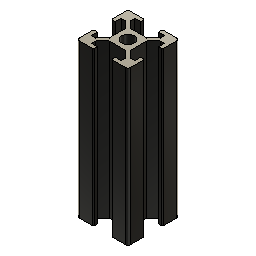
Support_Arm_ Assembly v9 (Autodesk Fusion 360 archive; units mm, degrees)
design "2020 Extrusion 60mm"
Autodesk Fusion 360 part; units mm, degrees
sketch "Sketch1" plane through (0, 0, 0) normal (0, 0, 1) x (1, 0, 0)
  line L0 (0, 1) -> (0, 6.1503)
  line L1 (1, 0) -> (6.15, 0)
  line L2 (0.3536, 6.5038) -> (1.5038, 6.5038)
  line L3 (1.5038, 6.5038) -> (1.5038, 4.2038)
  line L4 (1.5038, 4.2038) -> (3.2139, 4.2038)
  line L5 (3.2139, 4.2038) -> (5.804, 6.7939)
  line L6 (6.5036, 0.3536) -> (6.5036, 1.5036)
  line L7 (6.5036, 1.5036) -> (4.2036, 1.5036)
  line L8 (4.2036, 1.5036) -> (4.2036, 3.2136)
  line L9 (4.2036, 3.2136) -> (6.7937, 5.8037)
  line L10 (0, 6.1503) -> (0.3536, 6.5038)
  line L11 (6.15, 0) -> (6.5036, 0.3536)
  circle A0 centre (10, 10) radius 2.45
  line L12 (10, 10) -> (0, 0) construction
  line L13 (0, 19) -> (0, 13.85)
  line L14 (1, 20) -> (6.15, 20)
  line L15 (0, 13.85) -> (0.3536, 13.4964)
  line L16 (0, 13.85) -> (0.5, 13.85) construction
  line L17 (0.3536, 13.4964) -> (1.5036, 13.4964)
  line L18 (1.5036, 13.4964) -> (1.5036, 15.7964)
  line L19 (0, 20) -> (10, 10) construction
  line L20 (5.804, 6.7939) -> (5.804, 13.2061)
  line L21 (5.804, 13.2061) -> (3.2139, 15.7962)
  line L22 (1.5036, 15.7964) -> (3.2139, 15.7962)
  line L23 (6.15, 20) -> (6.5036, 19.6464)
  line L24 (6.15, 20) -> (6.65, 20) construction
  line L25 (6.5036, 19.6464) -> (6.5036, 18.4964)
  line L26 (6.5036, 18.4964) -> (4.2036, 18.4964)
  line L27 (4.2036, 18.4964) -> (4.2036, 16.7864)
  line L28 (4.2036, 16.7864) -> (6.7937, 14.1963)
  line L29 (10, 10) -> (20, 20) construction
  line L30 (10, 10) -> (20, 0) construction
  line L31 (19, 20) -> (13.85, 20)
  line L32 (20, 19) -> (20, 13.85)
  line L33 (13.85, 20) -> (13.4964, 19.6464)
  line L34 (13.85, 20) -> (14.35, 20) construction
  line L35 (13.4964, 19.6464) -> (13.4964, 18.4964)
  line L36 (20, 13.85) -> (19.6464, 13.4964)
  line L37 (20, 13.85) -> (20.5, 13.85) construction
  line L38 (19.6464, 13.4964) -> (18.4964, 13.4964)
  line L39 (13.4964, 18.4964) -> (15.7964, 18.4964)
  line L40 (18.4964, 13.4964) -> (18.4964, 15.7964)
  line L41 (15.7964, 18.4964) -> (15.7964, 16.7864)
  line L42 (15.7964, 16.7864) -> (13.2064, 14.1963)
  line L43 (13.2064, 14.1963) -> (6.7937, 14.1963)
  line L44 (18.4964, 15.7964) -> (16.7864, 15.7964)
  line L45 (16.7864, 15.7964) -> (14.1963, 13.2063)
  line L46 (19, 0) -> (13.85, 0)
  line L47 (20, 1) -> (20, 6.15)
  line L48 (13.85, 0) -> (13.4964, 0.3536)
  line L49 (13.85, 0) -> (14.35, 0) construction
  line L50 (13.4964, 0.3536) -> (13.4964, 1.5036)
  line L51 (13.4964, 1.5036) -> (15.7964, 1.5036)
  line L52 (15.7964, 1.5036) -> (15.7964, 3.2136)
  line L53 (15.7964, 3.2136) -> (13.2063, 5.8037)
  line L54 (6.7937, 5.8037) -> (13.2063, 5.8037)
  line L55 (20, 6.15) -> (19.6464, 6.5036)
  line L56 (20, 6.15) -> (20.5, 6.15) construction
  line L57 (19.6464, 6.5036) -> (18.4964, 6.5036)
  line L58 (18.4964, 6.5036) -> (18.4964, 4.2036)
  line L59 (18.4964, 4.2036) -> (16.7864, 4.2036)
  line L60 (16.7864, 4.2036) -> (14.1963, 6.7937)
  line L61 (14.1963, 6.7937) -> (14.1963, 13.2063)
  arc A1 (0, 1) -> (1, 0) centre (1, 1) ccw
  arc A2 (1, 20) -> (0, 19) centre (1, 19) ccw
  arc A3 (20, 19) -> (19, 20) centre (19, 19) ccw
  arc A4 (19, 0) -> (20, 1) centre (19, 1) ccw
  dimension "d9" = 2.3
  dimension "d11" = 3.663
  dimension "d13" = 2.3
  dimension "d17" = 135
  dimension "d18" = 135
  dimension "d19" = 135
  dimension "d20" = 6.1503
  dimension "d21" = 1.1503
  dimension "d22" = 0.5
  dimension "d23" = 135
  dimension "d24" = 0.5
  dimension "d25" = 6.15
  dimension "d26" = 1.15
  dimension "d27" = 4.9
  dimension "d28" = 10
  dimension "d29" = 10
  dimension "d30" = 1.4
  dimension "d31" = 0.7
  dimension "d32" = 6.15
  dimension "d33" = 20
  dimension "d34" = 6.15
  dimension "d35" = 45
  dimension "d36" = 0.5
  dimension "d37" = 1.15
  dimension "d38" = 2.3
  dimension "d40" = 3.663
  dimension "d41" = 0.7
  dimension "d42" = 0.5
  dimension "d43" = 45
  dimension "d44" = 1.15
  dimension "d45" = 2.3
  dimension "d47" = 3.663
  dimension "d48" = 0.7
  dimension "d49" = 6.15
  dimension "d50" = 6.15
  dimension "d51" = 135
  dimension "d52" = 0.5
  dimension "d53" = 1.15
  dimension "d54" = 20
  dimension "d55" = 135
  dimension "d56" = 0.5
  dimension "d57" = 1.15
  dimension "d58" = 2.3
  dimension "d59" = 2.3
  dimension "d61" = 0.7
  dimension "d63" = 3.663
  dimension "d64" = 0.7
  dimension "d65" = 6.15
  dimension "d66" = 6.15
  dimension "d67" = 135
  dimension "d68" = 0.5
  dimension "d69" = 20
  dimension "d70" = 1.15
  dimension "d71" = 2.3
  dimension "d73" = 0.7
  dimension "d74" = 135
  dimension "d75" = 0.5
  dimension "d76" = 1.15
  dimension "d77" = 2.3
  dimension "d78" = 1.71
  dimension "d79" = 1
  dimension "d80" = 1
  dimension "d81" = 1
  dimension "d82" = 1
  dimension "d83" = 1
  dimension "d84" = 1
  constraint vertical L0
  constraint perpendicular L0 L1
  constraint horizontal L2
  constraint perpendicular L2 L3
  constraint perpendicular L3 L4
  constraint perpendicular L1 L6
  constraint perpendicular L6 L7
  constraint perpendicular L7 L8
  constraint equal L5 L9
  constraint coincident A0.centre L12.start
  constraint coincident L12.end origin
  constraint vertical L13
  constraint collinear L0 L13
  constraint perpendicular L13 L14
  constraint horizontal L16
  constraint horizontal L17
  constraint perpendicular L17 L18
  constraint parallel L18 L20
  constraint parallel L19 L21
  constraint horizontal L24
  constraint vertical L25
  constraint perpendicular L25 L26
  constraint perpendicular L26 L27
  constraint parallel L19 L28
  constraint perpendicular L19 L29
  constraint perpendicular L29 L30
  constraint horizontal L31
  constraint perpendicular L31 L32
  constraint horizontal L34
  constraint vertical L35
  constraint horizontal L37
  constraint horizontal L38
  constraint perpendicular L35 L39
  constraint perpendicular L38 L40
  constraint perpendicular L39 L41
  constraint perpendicular L28 L42
  constraint horizontal L43
  constraint perpendicular L40 L44
  constraint parallel L29 L45
  constraint horizontal L46
  constraint perpendicular L46 L47
  constraint horizontal L49
  constraint vertical L50
  constraint perpendicular L50 L51
  constraint perpendicular L51 L52
  constraint perpendicular L9 L53
  constraint horizontal L54
  constraint horizontal L56
  constraint horizontal L57
  constraint perpendicular L57 L58
  constraint perpendicular L58 L59
  constraint perpendicular L45 L60
  constraint vertical L61
  constraint tangent L1 A1
  constraint tangent L0 A1
  constraint coincident L19.start L14
  constraint coincident L19.start L13
  constraint tangent L14 A2
  constraint tangent L13 A2
  constraint coincident L29.end L31
  constraint coincident L29.end L32
  constraint tangent L31 A3
  constraint tangent L32 A3
  constraint coincident L30.end L47
  constraint coincident L30.end L46
  constraint tangent L47 A4
  constraint tangent L46 A4
  measures "d9" distance of L2.end L3.end
  measures "d11" distance of L4.end L5.end
  measures "d13" distance of L6.end L7.end
  measures "d17" angle of L4 L5
  measures "d18" angle of L8 L9
  measures "d19" angle of L2 L10
  measures "d20" distance of L12.end L0.end
  measures "d21" distance of L2.end L2.start
  measures "d22" distance of L0.end L2.start
  measures "d23" angle of L1 L11
  measures "d24" distance of L1.end L6.start
  measures "d25" distance of L12.end L1.end
  measures "d26" distance of L6.end L6.start
  measures "d27" diameter of A0
  measures "d28" vertical distance of L12.end A0.centre
  measures "d29" horizontal distance of L12.end A0.centre
  measures "d30" distance of L4.end L9
  measures "d31" distance of L4.end L12
  measures "d32" distance of L19.start L13.end
  measures "d33" distance of L12.end L19.start
  measures "d34" distance of L19.start L14.end
  measures "d35" angle of L15 L16
  measures "d36" distance of L13.end L15.end
  measures "d37" distance of L15.end L17.end
  measures "d38" distance of L17.end L18.end
  measures "d40" distance of L20.end L21.end
  measures "d41" distance of L19 L20.end
  measures "d42" distance of L14.end L23.end
  measures "d43" angle of L23 L24
  measures "d44" distance of L23.end L25.end
  measures "d45" distance of L25.end L26.end
  measures "d47" distance of L27.end L28.end
  measures "d48" distance of L19 L28.end
  measures "d49" distance of L29.end L31.end
  measures "d50" distance of L29.end L32.end
  measures "d51" angle of L33 L34
  measures "d52" distance of L31.end L33.end
  measures "d53" distance of L33.end L35.end
  measures "d54" distance of L19.start L29.end
  measures "d55" angle of L36 L37
  measures "d56" distance of L32.end L36.end
  measures "d57" distance of L36.end L38.end
  measures "d58" distance of L35.end L39.end
  measures "d59" distance of L38.end L40.end
  measures "d61" distance of L29 L42.end
  measures "d63" distance of L44.end L45.end
  measures "d64" distance of L29 L45.end
  measures "d65" distance of L30.end L46.end
  measures "d66" distance of L30.end L47.end
  measures "d67" angle of L48 L49
  measures "d68" distance of L46.end L48.end
  measures "d69" distance of L12.end L30.end
  measures "d70" distance of L48.end L50.end
  measures "d71" distance of L50.end L51.end
  measures "d73" distance of L30 L52.end
  measures "d74" angle of L55 L56
  measures "d75" distance of L47.end L55.end
  measures "d76" distance of L55.end L57.end
  measures "d77" distance of L57.end L58.end
  measures "d78" distance of L58.end L59.end
  measures "d79" radius of A1
  measures "d80" distance of L12.end L1.start
  measures "d81" distance of L12.end L0.start
  measures "d82" radius of A2
  measures "d83" radius of A3
  measures "d84" radius of A4
extrude "Extrude1" add sketch "Sketch1" along normal blind 60

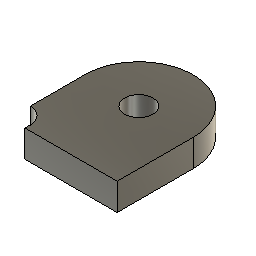
design "Arm travel stop left"
Autodesk Fusion 360 part; units mm, degrees
sketch "Sketch1" plane through (0, 0, 0) normal (0, 0, 1) x (1, 0, 0)
  line L0 (0, 0) -> (0, 14)
  line L1 (0, 0) -> (20, 0)
  line L2 (10, 0) -> (10, 14) construction
  line L3 (20, 0) -> (20, 14)
  arc A0 (20, 14) -> (0, 14) centre (10, 14) ccw
  circle A1 centre (10, 14) radius 2.6
  dimension "d1" = 14
  dimension "d2" = 20
  dimension "d3" = 14
  dimension "d4" = 14
  dimension "d5" = 5.2
  constraint coincident L0.start L1.start
  constraint vertical L0
  constraint horizontal L1
  constraint midpoint L1 L2.start
  constraint perpendicular L1 L2
  constraint perpendicular L1 L3
  constraint coincident L2.end A0.centre
  measures "d1" distance of L0.start L0.end
  measures "d2" distance of L0.start L1.end
  measures "d3" distance of L2.start L2.end
  measures "d4" distance of L1.end L3.end
  measures "d5" diameter of A1
extrude "Extrude1" add sketch "Sketch1" along normal blind 5
sketch "Sketch2" plane through (0, 0, 5) normal (0, 0, 1) x (-1, 0, 0)
  circle A0 centre (-10, -14) radius 2.6
  line L0 (0, 0) -> (-20, 0)
  line L1 (-20, 0) -> (-20, -14)
  arc A1 (-20, -14) -> (0, -14) centre (-10, -14) ccw
  line L2 (0, -14) -> (0, 0)
  circle A2 centre (-10, -14) radius 6 construction
  line L3 (-10, -14) -> (-5.7574, -9.7574) construction
  line L4 (-10, -14) -> (-4, -14) construction
  line L5 (-10, -14) -> (-14.2426, -9.7574) construction
  line L6 (-10, -14) -> (-14.2426, -18.2426) construction
  line L7 (-10, -14) -> (-5.7574, -18.2426) construction
  dimension "d8" = 12
  dimension "d9" = 45
  constraint concentric A0 A2
  constraint horizontal L4
  constraint coincident A0.centre A1.centre
  constraint coincident A2 L3.end
  constraint coincident A2 L5.end
  constraint perpendicular L3 L5
  constraint coincident A2 L6.end
  constraint perpendicular L5 L6
  constraint coincident A2 L7.end
  constraint perpendicular L6 L7
  measures "d8" diameter of A2
  measures "d9" angle of L3 L4
hole "Hole1" [suppressed]
sketch "Sketch3" plane through (0, 0, 0) normal (0, 0, -1) x (1, 0, 0)
  circle A0 centre (10, -14) radius 2.6
  line L0 (20, 0) -> (0, 0)
  line L1 (0, 0) -> (0, -14)
  arc A1 (0, -14) -> (20, -14) centre (10, -14) ccw
  line L2 (20, -14) -> (20, 0)
  circle A2 centre (10, -14) radius 10 construction
  line L3 (10, -24) -> (10, -4) construction
  point P0 (10, -7.875)
  dimension "d33" = 20
  dimension "d51" = 6.125
  constraint concentric A0 A2
  constraint midpoint A1 L3.start
  constraint coincident A2 L3.end
  constraint vertical L3
  constraint coincident L3 P0
  measures "d33" diameter of A2
  measures "d51" distance of A0.centre P0
hole "Hole5" [suppressed]
thread "Thread2" [suppressed]
sketch "Sketch7" plane through (0, 0, 0) normal (0, 0, -1) x (1, 0, 0)
  circle A0 centre (10, -14) radius 2.6
  line L0 (20, 0) -> (0, 0)
  line L1 (0, 0) -> (0, -14)
  arc A1 (0, -14) -> (20, -14) centre (10, -14) ccw
  line L2 (20, -14) -> (20, 0)
  line L3 (0, 0) -> (0, -4) construction
  line L4 (0, 0) -> (3, 0) construction
  line L5 (3, 0) -> (3, -1)
  arc A2 (0, -4) -> (3, -1) centre (0, -1) ccw
  dimension "d44" = 4
  dimension "d45" = 3
  dimension "d49" = 1
  dimension "d50" = 3
  constraint coincident L0.end L1.start
  constraint perpendicular L0 L3
  constraint perpendicular L3 L4
  constraint perpendicular L0 L5
  constraint tangent L5 A2
  measures "d44" distance of L0.end L3.end
  measures "d45" distance of L0.end L4.end
  measures "d49" distance of L4.end L5.end
  measures "d50" radius of A2
extrude "Extrude2" cut sketch "Sketch7" against normal blind 5 contours L0 L1 L5 A2

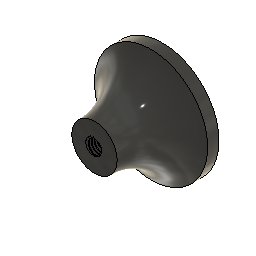
design "Pin_Release_Handle"
Autodesk Fusion 360 part; units mm, degrees
sketch "Sketch1" plane through (0, 0, 0) normal (0, 0, 1) x (1, 0, 0)
  line L0 (0, 0) -> (4, 0)
  line L1 (4, 0) -> (4, 12) construction
  line L2 (4, 0) -> (10, 0) construction
  line L3 (10, 0) -> (10, 10) construction
  line L4 (10, 0) -> (4, 0) construction
  line L5 (10, 10) -> (10, 12)
  line L6 (0, 0) -> (0, 12)
  line L7 (0, 12) -> (10, 12)
  arc A0 (10, 10) -> (4, 0) centre (15.3333, 0) ccw
  dimension "d1" = 4
  dimension "d2" = 12
  dimension "d5" = 90
  dimension "d7" = 12
  dimension "d9" = 2
  dimension "d10" = 6
  constraint coincident L0.start L6.start
  constraint horizontal L0
  constraint perpendicular L0 L1
  constraint perpendicular L1 L2
  constraint coincident L2.end L3.start
  constraint parallel L3 L5
  constraint perpendicular L0 L6
  constraint horizontal L7
  constraint tangent L1 A0
  measures "d1" distance of L0.start L0.end
  measures "d2" distance of L0.end L1.end
  measures "d5" angle of L3 L4
  measures "d7" distance of L0.start L6.end
  measures "d9" distance of L3.end L5.end
  measures "d10" distance of L0.end L2.end
revolve "Revolve2" add sketch "Sketch1" angle 360 about axis through (0, 0, 0) along (0, 1, 0)
sketch "Sketch2" plane through (0, 0, 0) normal (0, -1, 0) x (1, 0, 0)
  circle A0 centre (0, 0) radius 4
  constraint coincident A0.centre origin
hole "Hole1" at (0, 0, 0) direction (0, 1, 0) diameter 2.529 depth 7 tip angle 180
thread "Thread1" "ISO Metric profile 3.0 M3x0.5 6H" major diameter 3.086 minor diameter 2.529 pitch 0.5 angle 60 modelled right hand crest width 0.1368 on face at (0.1259, 2.3333, -1.2582) crest through (0, 0.125, -1.2645)

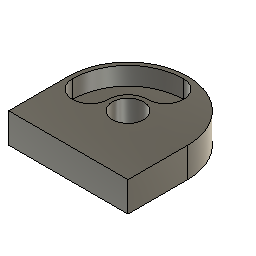
design "Alternate hindge stop left"
Autodesk Fusion 360 part; units mm, degrees
sketch "Sketch1" plane through (0, 0, 0) normal (0, 0, 1) x (1, 0, 0)
  line L0 (0, 0) -> (20, 0)
  line L1 (0, 0) -> (0, 10)
  line L2 (20, 0) -> (20, 10)
  line L3 (0, 10) -> (20, 10) construction
  arc A0 (20, 10) -> (0, 10) centre (10, 10) ccw
  circle A1 centre (10, 10) radius 2.6
  dimension "d1" = 20
  dimension "d2" = 10
  dimension "d3" = 10
  dimension "d4" = 5.2
  constraint coincident L0.start L1.start
  constraint horizontal L0
  constraint perpendicular L0 L1
  constraint perpendicular L0 L2
  constraint midpoint L3 A0.centre
  constraint concentric A0 A1
  measures "d1" distance of L0.start L0.end
  measures "d2" distance of L0.start L1.end
  measures "d3" distance of L0.end L2.end
  measures "d4" diameter of A1
extrude "Extrude1" add sketch "Sketch1" along normal blind 5
sketch "Sketch2" plane through (0, 0, 5) normal (0, 0, 1) x (-1, 0, 0)
  circle A0 centre (-10, -10) radius 2.6
  line L0 (0, 0) -> (-20, 0)
  line L1 (-20, 0) -> (-20, -10)
  arc A1 (-20, -10) -> (0, -10) centre (-10, -10) ccw
  line L2 (0, -10) -> (0, 0)
  line L3 (-10, -10) -> (-10, -20) construction
  line L4 (-10, -10) -> (0, -10) construction
  arc A2 (-10, -13.3) -> (-6.7, -10) centre (-10, -10) ccw
  arc A3 (-10, -19.3) -> (-0.7, -10) centre (-10, -10) ccw
  line L5 (-0.7, -10) -> (-6.7, -10) construction
  line L6 (-10, -19.3) -> (-10, -13.3) construction
  arc A4 (-10, -13.3) -> (-10, -19.3) centre (-10, -16.3) ccw
  arc A5 (-0.7, -10) -> (-6.7, -10) centre (-3.7, -10) ccw
  dimension "d11" = 6.3
  dimension "d12" = 3
  constraint coincident A0.centre A1.centre
  constraint midpoint A1 L3.end
  constraint coincident A1.end L2.start
  constraint coincident L3 A2.start
  constraint coincident L4 A2.end
  constraint coincident L3 A3.start
  constraint coincident L4 A3.end
  constraint midpoint L6 A4.centre
  constraint midpoint L5 A5.centre
  measures "d11" distance of A0.centre A4.centre
  measures "d12" radius of A4
extrude "Extrude2" cut sketch "Sketch2" against normal blind 3 contours A2 A3 A4 A5
